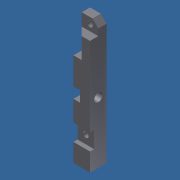
# Autodesk Inventor part: CHASSI ESQUERDO(37)
Saved by Autodesk Inventor 2012 SP1 (Build 160190100, 190)
## iProperties
Created: 2012-07-23
Part Number: CHASSI ESQUERDO(37)
Material: Carbon Steel
Document SubType Name: Modeling
Designer: bruno.silveira
Mass: 480.07 g
Surface Area: 130 cm^2
Volume: 61 cm^3
Density: 7.87 g/cm^3
Author: bruno.silveira
Autodesk Inventor part; units mm, degrees
ref_plane "YZ Plane" through (0, 0, 0) normal (1, 0, 0) x (0, 1, 0)
ref_plane "XZ Plane" through (0, 0, 0) normal (0, 1, 0) x (-1, 0, 0)
ref_plane "XY Plane" through (0, 0, 0) normal (0, 0, 1) x (1, 0, 0)
sketch "Sketch1" plane through (0, 0, 0) normal (0, 0, 1) x (1, 0, 0)
  line L0 (0, 0) -> (20, 0)
  line L1 (20, 0) -> (20, 20)
  line L2 (20, 20) -> (0, 20)
  line L3 (0, 20) -> (0, 0)
  dimension "d0" = 20
  dimension "d1" = 20
  constraints: 8 end point, 2 parallel, 1 horizontal, 1 perpendicular
  measures "d0" distance of L0.end L1.end
  measures "d1" distance of L1.end L2.end
extrude "Extrusion1" add sketch "Sketch1" along normal blind 152.5
sketch "Sketch2" plane through (0, 20, 0) normal (0, 1, 0) x (1, 0, 0)
  line L0 (0, -152.5) -> (20, -152.5) projected
  line L1 (0, 0) -> (0, -152.5) projected
  line L2 (0, -80) -> (8, -80)
  line L3 (8, -80) -> (8, -67)
  line L4 (8, -67) -> (0, -67)
  line L5 (0, -67) -> (0, -80)
  dimension "d4" = 13
  dimension "d5" = 72.5
  dimension "d6" = 8
  constraints: 8 end point, 2 parallel, 1 horizontal, 1 perpendicular, 1 point on line
  measures "d4" distance of L4.end L2.start
  measures "d5" distance between parallel lines of L0 L2
  measures "d6" distance between parallel lines of L1 L3
extrude "Extrusion2" cut sketch "Sketch2" against normal blind 20
sketch "Sketch7" plane through (0, 0, 0) normal (-1, 0, 0) x (0, 0, 1)
  line L0 (0, 20) -> (0, 0) projected
  line L1 (42, 5) -> (22, 5)
  line L2 (22, 5) -> (22, 0)
  line L3 (22, 0) -> (42, 0)
  line L4 (42, 0) -> (42, 5)
  line L5 (67, 0) -> (67, 20) projected
  line L6 (0, 20) -> (67, 20) projected
  line L7 (0, 20) -> (0, 0) projected
  line L8 (0, 0) -> (67, 0) projected
  dimension "d40" = 20
  dimension "d41" = 22
  dimension "d90" = 5
  constraints: 8 end point, 2 parallel, 1 horizontal, 1 perpendicular, 1 point on line
  measures "d40" distance of L2.end L3.end
  measures "d41" distance between parallel lines of L0 L2
  measures "d90" distance between parallel lines of L3 L1
extrude "Extrusion5" cut sketch "Sketch7" against normal blind 20 contours L2 L1 L4 L3
sketch "Sketch12" plane through (0, 0, 152.5) normal (0, -1, 0) x (1, 0, 0)
  line L0 (20, -110.5) -> (20, 0) projected
  line L1 (20, 0) -> (0, 0) projected
  line L2 (0, -72.5) -> (0, 0) projected
  line L3 (0, -110.5) -> (0, -85.5) projected
  line L4 (20, -15) -> (0, -15)
  point P0 (0, -152.5)
  dimension "d91" = 15
  constraints: 2 end point, 2 point on line, 1 perpendicular
  measures "d91" distance between parallel lines of L4 L1
extrude "Extrusion6" cut sketch "Sketch12" against normal blind 10
sketch "Sketch13" plane through (0, 0, 80) normal (0, -1, 0) x (1, 0, 0)
  line L0 (0, 57.5) -> (10, 57.5)
  line L1 (10, 57.5) -> (10, 32.5)
  line L2 (10, 32.5) -> (0, 32.5)
  line L3 (0, 32.5) -> (0, 57.5)
  point P0 (0, -80)
  dimension "d94" = 25
  dimension "d95" = 10
  constraints: 8 end point, 2 parallel, 1 horizontal, 1 perpendicular
  measures "d94" distance of L2.end L0.start
  measures "d95" distance of L1.end L2.end
extrude "Extrusion7" cut sketch "Sketch13" against normal blind 10
chamfer "Chamfer5" distance 10 angle 45 1 edges at (10, 10, 125)
sketch "Sketch14" plane through (20, 0, 0) normal (1, 0, 0) x (0, 0, -1)
  line L0 (0, 20) -> (-152.5, 20) projected
  line L1 (-80, 20) -> (-80, 0) projected
  line L2 (-67, 20) -> (-67, 0) projected
  point P0 (-73.5, 10)
  dimension "d101" = 6.5
  dimension "d102" = 10
  measures "d101" distance from line of L1 point (-73.5, 10)
  measures "d102" distance from line of L0 point (-73.5, 10)
hole "Hole7" at (20, 10, 73.5) direction (-1, 0, 0) diameter 6.5 depth 13 tip angle 118 counterbore diameter 10 counterbore depth 7
chamfer "Chamfer6" distance 7 angle 45 1 edges at (20, 15, 152.5)
sketch "Sketch15" plane through (0, 20, 0) normal (0, 1, 0) x (1, 0, 0)
  line L0 (20, 0) -> (20, -145.5) projected
  line L1 (0, -152.5) -> (13, -152.5) projected
  point P0 (10, -145)
  dimension "d113" = 7.5
  dimension "d114" = 10
  measures "d113" distance from line of L1 point (10, -145)
  measures "d114" distance from line of L0 point (10, -145)
hole "Hole8" at (10, 20, 145) direction (0, -1, 0) diameter 6.5 depth 10 tip angle 118 counterbore diameter 10 counterbore depth 7
sketch "Sketch16" plane through (0, 20, 0) normal (0, 1, 0) x (1, 0, 0)
  line L0 (20, 0) -> (20, -145.5) projected
  line L1 (0, -22) -> (20, -22) projected
  line L2 (0, -42) -> (20, -42) projected
  point P0 (10, -32)
  dimension "d122" = 10
  dimension "d123" = 10
  measures "d122" distance from line of L2 point (10, -32)
  measures "d123" distance from line of L0 point (10, -32)
hole "Hole9" at (10, 20, 32) direction (0, -1, 0) diameter 6.5 depth 15 tip angle 118 counterbore diameter 10 counterbore depth 7
sketch "Sketch17" plane through (0, 0, 0) normal (-1, 0, 0) x (0, 0, 1)
  line L0 (0, 20) -> (67, 20) projected
  line L1 (28.75, 5) -> (28.75, 13) projected
  line L2 (35.25, 5) -> (35.25, 13) projected
  line L3 (37, 13) -> (27, 13) projected
  line L4 (42, 5) -> (42, 0) projected
  line L5 (42, 0) -> (67, 0) projected
  line L6 (67, 0) -> (67, 20) projected
  line L7 (0, 20) -> (67, 20) projected
  line L8 (0, 20) -> (0, 0) projected
  line L9 (0, 0) -> (22, 0) projected
  line L10 (22, 0) -> (22, 5) projected
  line L11 (22, 5) -> (42, 5) projected
  line L12 (37, 13) -> (37, 20) projected
  line L13 (27, 13) -> (27, 20) projected
  line L14 (32, 5) -> (32, 20)
  point P0 (39.5, 10)
  point P1 (24.5, 10)
  dimension "d131" = 15
  dimension "d132" = 7.5
  dimension "d133" = 10
  constraints: 2 end point, 1 midpoint, 1 perpendicular, 1 point on line
  measures "d131" distance of point (39.5, 10) point (24.5, 10)
  measures "d132" horizontal distance of L14.start point (39.5, 10)
  measures "d133" distance from line of L0 point (24.5, 10)
hole "Hole10" at (0, 10, 39.5) at (0, 10, 24.5) direction (1, 0, 0) diameter 3.2 depth 12 tip angle 118
sketch "Sketch18" plane through (0, 0, 0) normal (0, 0, -1) x (-1, 0, 0)
  line L0 (0, 0) -> (-20, 0) projected
  line L1 (-20, 0) -> (-20, 20) projected
  point P0 (-13, 10)
  dimension "d141" = 7
  dimension "d142" = 10
  measures "d141" distance from line of L1 point (-13, 10)
  measures "d142" distance from line of L0 point (-13, 10)
hole "Hole11" at (13, 10, 0) direction (0, 0, 1) diameter 4.917 depth 8 tip angle 118 thread size "M6x1" class "6H" standard "ANSI Metric M Profile"
chamfer "Chamfer7" distance 0.5 angle 45 1 edges at (13, 7.5415, 0)
sketch "Sketch19" plane through (0, 0, 0) normal (-1, 0, 0) x (0, 0, 1)
  line L0 (0, 20) -> (0, 0) projected
  line L1 (0, 0) -> (22, 0) projected
  point P0 (6.5, 10)
  dimension "d153" = 6.5
  dimension "d154" = 10
  measures "d153" distance from line of L0 point (6.5, 10)
  measures "d154" distance from line of L1 point (6.5, 10)
hole "Hole12" at (0, 10, 6.5) direction (1, 0, 0) diameter 4.917 depth 8 tip angle 118 thread size "M6x1" class "6H" standard "ANSI Metric M Profile"
chamfer "Chamfer8" distance 0.5 angle 45 1 edges at (0, 10, 4.0415)
body "Solid1"
